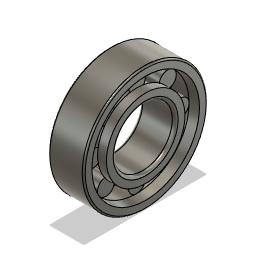
old-Bearing_GOST_8328-75_2000 (Autodesk Fusion 360 design; units mm, degrees)
Autodesk Fusion 360 part; units mm, degrees
sketch "Sketch1" plane through (0, 0, 0) normal (0, 0, 1) x (1, 0, 0)
  line L0 (-124.2305, 0) -> (125.7695, 0)
  line L1 (-6, 10) -> (6, 10)
  line L2 (-6, 10) -> (-6, 13.3)
  line L3 (-6, 13.3) -> (-3, 13.3)
  line L4 (6, 10) -> (6, 13.3)
  line L5 (6, 13.3) -> (3, 13.3)
  line L6 (3, 13.3) -> (3, 11.97)
  line L7 (3, 11.97) -> (-3, 11.97)
  line L8 (-3, 11.97) -> (-3, 13.3)
  line L9 (-3, 17.7) -> (3, 17.7)
  line L10 (3, 17.7) -> (6, 18.229)
  line L11 (-3, 17.7) -> (-6, 18.229)
  line L12 (-6, 18.229) -> (-6, 21)
  line L13 (-6, 21) -> (6, 21)
  line L14 (6, 21) -> (6, 18.229)
  line L15 (-3, 17.7) -> (-3, 13.3)
  line L16 (3, 17.7) -> (3, 13.3)
  line L17 (-3, 14.835) -> (3, 14.835)
  point P0 (0, 11.97)
  dimension "d37" = 12
  dimension "d38" = 20
  dimension "d39" = 3
  dimension "d40" = 23.94
  dimension "d41" = 26.6
  dimension "d42" = 35.4
  dimension "d43" = 10
  dimension "d44" = 10
  dimension "d45" = 42
  dimension "d47" = 2.865
  constraint horizontal L0
  constraint horizontal origin L0.start
  constraint horizontal L1
  constraint perpendicular L1 L2
  constraint perpendicular L2 L3
  constraint perpendicular L1 L4
  constraint perpendicular L4 L5
  constraint perpendicular L5 L6
  constraint perpendicular L4 L7
  constraint perpendicular L3 L8
  constraint equal L3 L5
  constraint midpoint L7 P0
  constraint vertical origin P0
  constraint horizontal L3.end L5.end
  constraint horizontal L9
  constraint vertical L3.end L9.start
  constraint vertical L5.end L9.end
  constraint vertical L2.end L11.end
  constraint vertical L4.end L10.end
  constraint vertical L12
  constraint perpendicular L12 L13
  constraint perpendicular L13 L14
  constraint coincident L15 L17.start
  constraint perpendicular L15 L17
  measures "d37" distance of L1.start L1.end
  measures "d39" distance of L4 L6
  measures "d43" angle of L9 L10
  measures "d44" angle of L9 L11
  measures "d47" distance of L7 L17
revolve "Revolve3" add sketch "Sketch1" angle 360 about axis through (-124.2305, 0, 0) along (1, 0, 0) contours L1 L2 L3 L4 L5 L6 L7 L8 | L9 L10 L11 L12 L13 L14 makes body 1 at (2, 9.9503, -0.9957) makes body 2 at (2, 20.8956, -2.0909)
revolve "Revolve4" add sketch "Sketch1" angle 360 about axis through (-3, 14.835, 0) along (1, 0, 0) separate body contours L9 L15 L16 L17 makes body 3
pattern_circular "C-Pattern2" count 8 over 360 about axis through (-6, 0, 0) along (1, 0, 0) of bodies 3 makes body 4 at (-1, 12.6142, 12.4123) makes body 5 at (-1, 0.1428, 17.6964) makes body 6 at (-1, -12.4123, 12.6142) makes body 7 at (-1, -17.6964, 0.1428) makes body 8 at (-1, -12.6142, -12.4123) makes body 9 at (-1, -0.1428, -17.6964) makes body 10 at (-1, 12.4123, -12.6142)
fillet "Fillet3" radius 1 2 edges at (6, -3.6162, 9.3233) (-6, -3.6162, 9.3233) on bodies 1
fillet "Fillet4" radius 0.5 2 edges at (6, -7.5939, 19.5789) (-6, -7.5939, 19.5789) on bodies 2
equation "d = 20 mm"
equation "D = 42 mm"
equation "B = 12 mm"
equation "_r = 1 mm"
equation "_r1 = 0.5 mm"
equation "ADA = B * 0.25"
equation "BID1 = d + ( D - d ) / 3.333333"
equation "KAD1 = BID1 + 1.33333 * ( D - d ) / 3.3333333"
equation "KID1 = BID1 / 1.1111111111"
equation "d37 = B"
equation "d38 = d"
equation "d39 = ADA"
equation "d40 = KID1"
equation "d41 = BID1"
equation "d42 = KAD1"
equation "d45 = D"
equation "d47 = ( KAD1 - KID1 ) * 0.5 * 0.5"
equation "CylCount = round(PI * ( KID1 + 0.5 * ( KAD1 - KID1 ) ) / ( ( KAD1 - KID1 ) / 2 ) / 2)"
equation "d52 = CylCount"
equation "d55 = _r"
equation "d57 = _r1"
